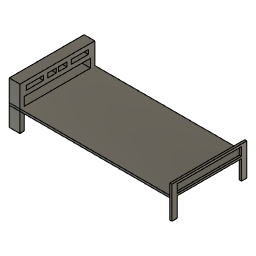
frame v3 (Autodesk Fusion 360 design; units mm, degrees)
Autodesk Fusion 360 part; units mm, degrees
sketch "Sketch1" plane through (0, 0, 0) normal (1, 0, 0) x (0, 1, 0)
  line L0 (0, 0) -> (0, 200)
  line L1 (0, 200) -> (350, 200)
  line L2 (350, 200) -> (350, 0)
  line L3 (350, 0) -> (330, 0)
  line L4 (330, 0) -> (330, 90)
  line L5 (330, 90) -> (20, 90)
  line L6 (20, 90) -> (20, 0)
  line L7 (20, 190) -> (20, 150)
  line L8 (20, 150) -> (330, 150)
  line L9 (330, 150) -> (330, 190)
  line L10 (330, 190) -> (20, 190)
  line L11 (30, 180) -> (30, 160)
  line L12 (30, 160) -> (110, 160)
  line L13 (110, 160) -> (110, 180)
  line L14 (110, 180) -> (30, 180)
  line L15 (320, 180) -> (240, 180)
  line L16 (240, 180) -> (240, 160)
  line L17 (240, 160) -> (320, 160)
  line L18 (320, 160) -> (320, 180)
  line L19 (130, 180) -> (130, 160)
  line L20 (130, 160) -> (170, 160)
  line L21 (170, 160) -> (170, 180)
  line L22 (170, 180) -> (130, 180)
  line L23 (220, 180) -> (220, 160)
  line L24 (220, 160) -> (180, 160)
  line L25 (180, 160) -> (180, 180)
  line L26 (180, 180) -> (220, 180)
  line L27 (20, 140) -> (20, 100)
  line L28 (20, 100) -> (330, 100)
  line L29 (330, 100) -> (330, 140)
  line L30 (330, 140) -> (20, 140)
  line L31 (20, 0) -> (0, 0)
  constraint coincident L0.start L31.end
  constraint vertical L0
  constraint perpendicular L0 L1
  constraint perpendicular L1 L2
  constraint perpendicular L2 L3
  constraint perpendicular L3 L4
  constraint perpendicular L2 L5
  constraint perpendicular L5 L6
  constraint perpendicular L1 L7
  constraint perpendicular L0 L8
  constraint perpendicular L8 L9
  constraint perpendicular L0 L10
  constraint perpendicular L10 L11
  constraint perpendicular L11 L12
  constraint perpendicular L12 L13
  constraint perpendicular L13 L14
  constraint perpendicular L13 L15
  constraint perpendicular L15 L16
  constraint perpendicular L13 L17
  constraint perpendicular L15 L18
  constraint perpendicular L14 L19
  constraint perpendicular L19 L20
  constraint perpendicular L20 L21
  constraint perpendicular L19 L22
  constraint perpendicular L22 L23
  constraint perpendicular L23 L24
  constraint perpendicular L24 L25
  constraint perpendicular L23 L26
  constraint perpendicular L8 L27
  constraint perpendicular L27 L28
  constraint perpendicular L28 L29
  constraint perpendicular L29 L30
  constraint perpendicular L0 L31
extrude "Extrude1" add sketch "Sketch1" along normal blind 50 contours L0 L1 L2 L3 L4 L5 L6 L31 | L7 L8 L9 L10 makes body 1
sketch "Sketch2" plane through (0, 0, 0) normal (1, 0, 0) x (0, 1, 0)
  line L0 (20, 100) -> (20, 90)
  line L1 (330, 100) -> (350, 100)
  line L2 (350, 100) -> (350, 90)
  line L3 (350, 90) -> (310, 90)
  line L4 (310, 90) -> (0, 90)
  line L5 (0, 90) -> (0, 100)
  line L6 (0, 100) -> (330, 100)
  constraint vertical L0
  constraint horizontal L1
  constraint perpendicular L1 L2
  constraint perpendicular L2 L3
  constraint perpendicular L0 L4
  constraint perpendicular L4 L5
  constraint perpendicular L0 L6
surface "Extrude2" add extruded along (1, 0, 0) between 0 and 750 path "Sketch2" along L2 L3 L4 L5 L6 L1 separate body makes body 2
ref_plane "WorkPlane1" through (750, 0, 0) normal (1, 0, 0) x (0, 1, 0)
sketch "Sketch3" plane through (750, 0, 0) normal (1, 0, 0) x (0, 1, 0)
  line L0 (350, 0) -> (350, 150)
  line L1 (350, 150) -> (0, 150)
  line L2 (0, 150) -> (0, 0)
  line L3 (0, 0) -> (25, 0)
  line L4 (25, 0) -> (25, 90.7963)
  line L5 (25, 90.7963) -> (325, 90.7963)
  line L6 (325, 90.7963) -> (325, 0)
  line L7 (325, 0) -> (350, 0)
  line L8 (325, 139.3791) -> (325, 100)
  line L9 (325, 100) -> (25, 100)
  line L10 (325, 139.3791) -> (25, 139.3791)
  line L11 (25, 139.3791) -> (25, 100)
  constraint vertical L0
  constraint perpendicular L0 L1
  constraint coincident L2.end L3.start
  constraint perpendicular L1 L2
  constraint perpendicular L2 L3
  constraint perpendicular L3 L4
  constraint perpendicular L4 L5
  constraint perpendicular L3 L6
  constraint perpendicular L0 L7
  constraint perpendicular L1 L8
  constraint perpendicular L8 L9
  constraint perpendicular L8 L10
  constraint perpendicular L9 L11
extrude "Extrude3" add sketch "Sketch3" along normal blind 10 separate body makes body 3
